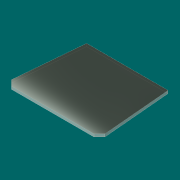
# Autodesk Inventor part: mirrorSides
Saved by Autodesk Inventor 2016 (Build 200138000, 138)
## iProperties
Created: 2015-10-14
Part Number: mirrorSides
Material: Glass
Document SubType Name: Modeling
Designer: Sawaiz
Density: 2.18 g/cm^3
Appearance: Clear
Author: Sawaiz
Autodesk Inventor part; units mm, degrees
ref_plane "YZ Plane" through (0, 0, 0) normal (1, 0, 0) x (0, 1, 0)
ref_plane "XZ Plane" through (0, 0, 0) normal (0, 1, 0) x (-1, 0, 0)
ref_plane "XY Plane" through (0, 0, 0) normal (0, 0, 1) x (1, 0, 0)
sketch "Sketch1" plane through (0, 0, 0) normal (0, 0, 1) x (1, 0, 0)
  line L0 (-37.1597, -43.7763) -> (-37.1597, 43.7763)
  line L1 (-37.1597, 43.7763) -> (43.1218, 50.8)
  line L2 (43.1218, 50.8) -> (43.1218, -50.8)
  line L3 (43.1218, -50.8) -> (-37.1597, -43.7763)
  line L4 (-37.1597, -43.7763) -> (43.1218, 50.8) construction
  line L5 (-37.1597, 43.7763) -> (43.1218, -50.8) construction
  point P0 (0, 0)
  dimension "d0" = 85
  dimension "d1" = 101.6
  dimension "d2" = 80.2815
  dimension "d5" = 87.5526
  constraints: 12 end point, 2 point on line, 1 equal length, 1 parallel, 1 vertical
  measures "d0" angle of L2 L1
  measures "d1" distance of L1.end L2.end
  measures "d2" distance between parallel lines of L2 L0
  measures "d5" distance of L0.start L0.end
extrude "Extrusion1" add sketch "Sketch1" along normal blind 3
sketch "Sketch4" plane through (0, 0, 3) normal (0, 0, 1) x (1, 0, 0)
  line L0 (-37.1597, 43.7763) -> (-37.1597, -43.7763) projected
  line L1 (-37.1597, -43.7763) -> (43.1218, -50.8) projected
  line L2 (43.1218, -50.8) -> (43.1218, 50.8) projected
  line L3 (43.1218, 50.8) -> (-37.1597, 43.7763) projected
  line L4 (43.1218, -50.8) -> (43.1218, 50.8) projected
  line L5 (43.1218, -44.45) -> (36.7718, -50.8)
  line L6 (36.7718, -50.8) -> (43.1218, -50.8)
  line L7 (43.1218, -50.8) -> (43.1218, -44.45)
  line L8 (43.1218, 50.8) -> (36.7718, 50.8)
  line L9 (36.7718, 50.8) -> (43.1218, 44.45)
  line L10 (43.1218, 50.8) -> (43.1218, 44.45)
  point P0 (0, 0)
  dimension "d9" = 6.35
  dimension "d10" = 6.35
  dimension "d11" = 45
  dimension "d12" = 45
  constraints: 12 end point, 2 collinear, 2 horizontal, 2 point on line
  measures "d9" distance of L2.end L9.end
  measures "d10" distance of L5.start L1.end
  measures "d11" angle of L2 L5
  measures "d12" angle of L2 L9
extrude "Extrusion3" cut sketch "Sketch4" against normal through all contours L9 L8 L3 | L3 L2 L9 | L5 L2 L1 | L1 L6 L5
equation "\"d1\" = height"
equation "\"d3\" = mirrorThickness"
equation "\"d9\" = fresnelMirrorChamfer"
equation "\"d10\" = fresnelMirrorChamfer"
equation "\"acrylicThickness\" = 6.35"
equation "\"height\" = 101.6"
equation "\"width\" = 101.6"
equation "\"depth\" = 101.6"
equation "\"mirrorAngle\" = 5deg"
equation "\"detectorWidth\" = 52"
equation "\"detectorHeight\" = 52"
equation "\"mirrorThickness\" = 3"
equation "\"fresnelThickness\" = 0.1"
equation "\"focalLength\" = 76.2"
equation "\"ior\" = 1.49"
equation "\"centerThickness\" = 1.524"
equation "\"fresnelAngle\" = 90deg"
equation "\"fresnelEffectiveDiameter\" = 76.2"
equation "\"mirrorSuppourtWidth\" = 38.1"
equation "\"sensorHolderORingID\" = 203.2"
equation "\"sensorHolderHeight\" = 88.9"
equation "\"oRingWidth\" = 3.175"
equation "\"sensorHolderSensorWidth\" = 53.975"
equation "\"sensorHolderFlushORingID\" = 304.8"
equation "\"sensorHolderWidth\" = 88.9"
equation "\"sensorHolderSensorHeight\" = 53.975"
equation "\"backGrooveBit\" = 4.8006"
equation "\"frontBackORingID\" = 419.1"
equation "\"mirrorGroove\" = 19.05"
equation "\"backMirrorGroove\" = 6.35"
equation "\"fresnelChamfer\" = 6.35"
equation "\"mirrorGrooveMill\" = 3.175"
equation "\"fresnelMirrorChamfer\" = 6.35"
equation "\"detectorOpeningWidth\" = 76.2"
equation "\"detectorOpeningHeight\" = 76.2"
body "Solid1"
